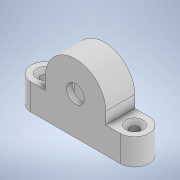
# Autodesk Inventor part: Крышка стойки подшипника
Saved by Autodesk Inventor 2020 (Build 240168000, 168)
## iProperties
Created: 2021-04-13
Part Number: Крышка стойки подшипника
Material: Типовые
Document SubType Name: Обычные детали
Designer: Антон
Density: 1 g/cm^3
Appearance: По умолчанию
Mass: 2.60501 g
Surface Area: 26.0903 cm^2
Volume: 2.60501 cm^3
Author: Антон
Autodesk Inventor part; units mm, degrees
ref_plane "YZ Plane" through (0, 0, 0) normal (1, 0, 0) x (0, 1, 0)
ref_plane "XZ Plane" through (0, 0, 0) normal (0, 1, 0) x (-1, 0, 0)
ref_plane "XY Plane" through (0, 0, 0) normal (0, 0, 1) x (1, 0, 0)
sketch "Эскиз2" plane through (0, 0, 0) normal (0, 0, 1) x (1, 0, 0)
  line L0 (0, 0) -> (10.05, 0)
  line L1 (10.05, 0) -> (10.05, 3.4)
  line L2 (10.05, 3.4) -> (0, 3.4)
  line L3 (0, 3.4) -> (0, 0)
  line L4 (10.05, 0) -> (31.15, 0)
  line L5 (31.15, 0) -> (31.15, 18.1)
  line L6 (31.15, 18.1) -> (10.05, 18.1)
  line L7 (10.05, 18.1) -> (10.05, 0)
  line L8 (31.15, 0) -> (41.2, 0)
  line L9 (41.2, 0) -> (41.2, 3.4)
  line L10 (41.2, 3.4) -> (31.15, 3.4)
  line L11 (31.15, 3.4) -> (31.15, 0)
  line L12 (20.6, 18.1) -> (20.6, 7.55)
  circle A0 centre (20.6, 7.55) radius 8.55
  line L13 (7, 0) -> (26, 0)
  line L14 (12.05, 7.55) -> (29.15, 7.55)
  line L15 (29.15, 7.55) -> (29.15, 0)
  line L16 (29.15, 0) -> (12.05, 0)
  line L17 (12.05, 0) -> (12.05, 7.55)
  point P0 (31.15, 3.4)
  point P1 (16.5875, 0)
  point P2 (24.6125, 0)
  point P3 (12.05, 0)
  point P4 (12.05, 7.55)
  point P5 (29.15, 0)
  dimension "d14" = 17.1
  dimension "d0" = 10.05
  dimension "d1" = 21.1
  dimension "d2" = 18.1
  dimension "d3" = 3.4
  dimension "d4" = 10.05
  dimension "d13" = 10.55
  dimension "d15" = 3.4
  constraints: 36 end point, 8 parallel, 4 horizontal, 4 perpendicular, 2 midpoint, 1 coincident, 1 collinear, 1 point on line, 1 vertical, 3 other
  measures "d0" distance of L2.end L1.end
  measures "d1" distance of L6.end L5.end
  measures "d2" distance of L5.end L4.end
  measures "d3" distance between parallel lines of L2 L0
  measures "d4" distance of L10.end L9.end
  measures "d13" distance of L12.end L12.start
  measures "d15" distance between parallel lines of L8 L10
extrude "Выдавливание1" add sketch "Эскиз2" along normal blind 6.1 contours L3 L2 L1 L0 | L1 L7 L6 L12 A0 L17 L4 | L6 L5 L4 L15 A0 L12 | L10 L9 L8 L5
sketch "Эскиз4" plane through (0, 0, 6.1) normal (0, 0, 1) x (1, 0, 0)
  line L0 (0, 0) -> (12.05, 0) projected
  line L1 (12.05, 0) -> (12.05, 7.55) projected
  arc A0 (29.15, 7.55) -> (12.05, 7.55) centre (20.6, 7.55) ccw projected
  line L2 (29.15, 7.55) -> (29.15, 0) projected
  line L3 (41.2, 0) -> (41.2, 3.4) projected
  line L4 (41.2, 3.4) -> (31.15, 3.4) projected
  line L5 (31.15, 3.4) -> (31.15, 18.1) projected
  line L6 (31.15, 18.1) -> (10.05, 18.1) projected
  line L7 (10.05, 18.1) -> (10.05, 3.4) projected
  line L8 (10.05, 3.4) -> (0, 3.4) projected
  line L9 (0, 3.4) -> (0, 0) projected
  line L10 (12.05, 0) -> (29.15, 0)
  line L11 (29.15, 0) -> (41.2, 0) projected
  constraints: 2 end point
extrude "Выдавливание3" add sketch "Эскиз4" along normal blind 2
ref_plane "РабПлоскость1" through (0, 0, 3.05) normal (0, 0, 1) x (1, 0, 0)
mirror "Зеркальное отражение2" about plane through (0, 0, 3.05) normal (0, 0, 1) of "Выдавливание3"
fillet "Сопряжение2" radius 10.55 2 edges at (31.15, 18.1, 3.05) (10.05, 18.1, 3.05)
sketch "Эскиз6" plane through (31.15, 3.4, 8.1) normal (0, 1, 0) x (1, 0, 0)
  line L0 (10.05, 10.1) -> (10.05, 0) projected
  line L1 (10.05, 5.05) -> (0, 5.05)
  line L2 (0, 10.1) -> (0, 0) projected
  line L3 (-21.1, 10.1) -> (-21.1, 0) projected
  line L4 (-21.1, 5.05) -> (-31.15, 5.05)
  line L5 (-31.15, 0) -> (-31.15, 10.1) projected
  line L6 (-26.125, 5.05) -> (-26.1, 5.05)
  line L7 (5.025, 5.05) -> (5, 5.05)
  point P0 (-31.15, 8.1)
  dimension "d35" = 0.025
  dimension "d36" = 0.025
  constraints: 8 end point, 6 midpoint, 2 coincident, 2 point on line
  measures "d35" distance of L6.start L6.end
  measures "d36" distance of L7.start L7.end
hole "Отверстие2" at (5.05, 3.4, 3.05) at (36.15, 3.4, 3.05) direction (0, -1, 0) diameter 3.2 end through all countersink diameter 6 countersink angle 90
sketch "Эскиз7" plane through (0, 0, 8.1) normal (0, -1, 0) x (1, 0, 0)
  line L0 (0, -10.1) -> (0, 0) projected
  line L1 (41.2, -10.1) -> (31.15, -10.1) projected
  line L2 (0, 0) -> (41.2, 0)
  line L3 (41.2, 0) -> (41.2, -10.1)
  line L4 (41.2, -10.1) -> (0, -10.1)
  line L5 (0, -10.1) -> (0, 0)
  line L6 (0, 0) -> (2, 0)
  line L7 (2, 0) -> (2, -2)
  line L8 (2, -2) -> (39.2, -2)
  line L9 (39.2, -2) -> (39.2, -8.1)
  line L10 (39.2, -8.1) -> (2, -8.1)
  line L11 (2, -8.1) -> (2, -2)
  line L12 (41.2, -10.1) -> (41.2, 0) projected
  line L13 (41.2, -10.1) -> (39.2, -10.1)
  line L14 (39.2, -10.1) -> (39.2, -8.1)
  point P0 (0, -8.1)
  dimension "d37" = 2
  dimension "d38" = 2
  dimension "d39" = 2
  dimension "d40" = 2
  constraints: 24 end point, 4 parallel, 4 perpendicular, 2 horizontal, 2 point on line
  measures "d37" distance of L0.end L6.end
  measures "d38" distance of L6.end L7.end
  measures "d39" distance of L1.start L13.end
  measures "d40" distance of L13.end L9.end
extrude "Выдавливание4" add sketch "Эскиз7" along normal blind 5.75 contours L0 L2 L7 L11 L10 L14 L1 L4 | L2 L3 L1 L14 L9 L8 L7
sketch "Эскиз8" plane through (0, 0, 8.1) normal (0, 0, 1) x (1, 0, 0)
  arc A0 (31.15, 7.55) -> (10.05, 7.55) centre (20.6, 7.55) ccw projected
  point P0 (0, 0)
hole "Отверстие3" at (20.6, 7.55, 8.1) direction (0, 0, -1) diameter 6.2 end through all
fillet "Сопряжение3" radius 5.05 2 edges at (0, -1.175, 8.1) (0, -1.175, -2)
fillet "Сопряжение4" radius 5.05 2 edges at (41.2, -1.175, 8.1) (41.2, -1.175, -2)
fillet "Сопряжение5" radius 3.05 2 edges at (2, -2.875, 6.1) (2, -2.875, 0)
fillet "Сопряжение6" radius 3.05 2 edges at (39.2, -2.875, 0) (39.2, -2.875, 6.1)
equation "\"d0\" = d4"
equation "\"d15\" = d3"
equation "\"Радиус_гибки\" = Толщина"
equation "\"Ширина_просечки\" = Толщина"
equation "\"Глубина_просечки\" = 0.5 * Толщина"
equation "\"Размер_просечки\" = 4 * Толщина"
equation "\"Мин_остаток\" = 2 * Толщина"
equation "\"Радиус_перехода\" = Радиус_гибки"
equation "\"Радиус_Якоби\" = Толщина"
equation "\"Размер_зазора\" = Толщина"
equation "\"Толщина\" = 0.5"
